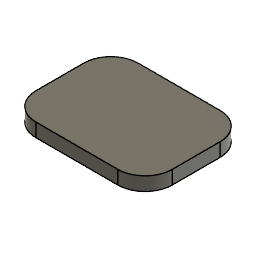
21_DAY- 3D Printable Mold (Autodesk Fusion 360 design; units mm, degrees)
part number: 2026-01-03-10-31-50-314
part number: 2026-01-03-10-33-35-516
part number: 2026-01-03-12-50-06-829
Autodesk Fusion 360 part; units mm, degrees
sketch "Sketch1" plane through (0, 0, 0) normal (0, 1, 0) x (1, 0, 0) in component "Key Chain"
  line L0 (0, 0) -> (50, 0)
  line L1 (50, 0) -> (50, 35)
  line L2 (50, 35) -> (0, 35)
  line L3 (0, 35) -> (0, 0)
  dimension "d1" = 50
  dimension "d2" = 35
  constraint horizontal L0
  constraint vertical L1
  constraint horizontal L2
  constraint vertical L3
  constraint coincident L0.start L3.end
  measures "d1" distance of L0.start L0.end
  measures "d2" distance of L0.start L2.end
extrude "Extrude1" add sketch "Sketch1" along normal blind 3 makes body 1 in component "Key Chain"
fillet "Fillet1" radius 7 4 edges at (0, 1.5, 0) (0, 1.5, -35) (50, 1.5, 0) (50, 1.5, -35) on bodies 1 in component "Key Chain"
sketch "Sketch2" plane through (0, 3, 0) normal (0, 1, 0) x (-1, 0, 0) in component "Key Chain"
  arc A0 (-50, -28) -> (-43, -35) centre (-43, -28) ccw
  line L0 (-43, -35) -> (-7, -35)
  arc A1 (-7, -35) -> (0, -28) centre (-7, -28) ccw
  line L1 (0, -28) -> (0, -7)
  arc A2 (0, -7) -> (-7, 0) centre (-7, -7) ccw
  line L2 (-7, 0) -> (-43, 0)
  arc A3 (-43, 0) -> (-50, -7) centre (-43, -7) ccw
  line L3 (-50, -7) -> (-50, -28)
  line L4 (-50, -17.5) -> (-45, -17.5) construction
  dimension "d7" = 5
  constraint midpoint L3 L4.start
  constraint perpendicular L3 L4
  measures "d7" distance of L4.start L4.end
hole "Hole1" at (45, 3, -17.5) direction (0, -1, 0) diameter 5 end up to surface (3 mm away) bodies 1 in component "Key Chain"
sketch "Sketch3" plane through (0, 3, 0) normal (0, 1, 0) x (-1, 0, 0) in component "Key Chain"
  circle A0 centre (-45, -17.5) radius 2.5
  arc A1 (-50, -28) -> (-43, -35) centre (-43, -28) ccw
  line L0 (-43, -35) -> (-7, -35)
  arc A2 (-7, -35) -> (0, -28) centre (-7, -28) ccw
  line L1 (0, -28) -> (0, -7)
  arc A3 (0, -7) -> (-7, 0) centre (-7, -7) ccw
  line L2 (-7, 0) -> (-43, 0)
  arc A4 (-43, 0) -> (-50, -7) centre (-43, -7) ccw
  line L3 (-50, -7) -> (-50, -28)
  line L4 (-3.7756, -4.293) -> (-42.3384, -4.293) construction
  line L5 (-42.3384, -4.293) -> (-42.3384, -31.526) construction
  line L6 (-42.3384, -31.526) -> (-3.7756, -31.526) construction
  line L7 (-3.7756, -31.526) -> (-3.7756, -4.293) construction
  dimension "d10" = 7
  text T0 "PIYUSH" font "Arial" height 7 bold align left middle in box 38.5628 x 27.233 at (-3.7756, -4.293) x (-1, 0) y (0, -1) spacing 1 kerned
extrude "Extrude2" add sketch "Sketch3" along normal blind 1 text T0 bodies 1 in component "Key Chain"
sketch "Sketch1 (2)" plane through (0, 3, 0) normal (0, 1, 0) x (-1, 0, 0) in component "One Part Mold"
  arc A0 (-50, -28) -> (-43, -35) centre (-43, -28) ccw
  line L0 (-43, -35) -> (-7, -35)
  arc A1 (-7, -35) -> (0, -28) centre (-7, -28) ccw
  line L1 (0, -28) -> (0, -7)
  arc A2 (0, -7) -> (-7, 0) centre (-7, -7) ccw
  line L2 (-7, 0) -> (-43, 0)
  arc A3 (-43, 0) -> (-50, -7) centre (-43, -7) ccw
  line L3 (-50, -7) -> (-50, -28)
  circle A4 centre (-45, -17.5) radius 2.5
  line L4 (-10.2551, -14.4095) -> (-10.2551, -21.4095)
  line L5 (-10.2551, -21.4095) -> (-11.6685, -21.4095)
  line L6 (-11.6685, -21.4095) -> (-11.6685, -14.4095)
  line L7 (-11.6685, -14.4095) -> (-10.2551, -14.4095)
  line L8 (-33.1269, -14.4095) -> (-33.1269, -21.4095)
  line L9 (-33.1269, -21.4095) -> (-34.5402, -21.4095)
  line L10 (-34.5402, -21.4095) -> (-34.5402, -18.6544)
  line L11 (-34.5402, -18.6544) -> (-37.3097, -18.6544)
  line L12 (-37.3097, -18.6544) -> (-37.3097, -21.4095)
  line L13 (-37.3097, -21.4095) -> (-38.723, -21.4095)
  line L14 (-38.723, -21.4095) -> (-38.723, -14.4095)
  line L15 (-38.723, -14.4095) -> (-37.3097, -14.4095)
  line L16 (-37.3097, -14.4095) -> (-37.3097, -17.4702)
  line L17 (-37.3097, -17.4702) -> (-34.5402, -17.4702)
  line L18 (-34.5402, -17.4702) -> (-34.5402, -14.4095)
  line L19 (-34.5402, -14.4095) -> (-33.1269, -14.4095)
  line L20 (-26.2415, -16.6871) -> (-27.6166, -16.8208)
  spline S0 degree 3 poles (-27.6166, -16.8208) (-27.6618, -16.6117) (-27.7446, -16.2287) (-28.0031, -15.9364) (-28.1204, -15.8038) knots 0 0 0 0 0.062919 0.115193 0.115193 0.115193 0.115193
  spline S1 degree 3 poles (-28.1204, -15.8038) (-28.2646, -15.7092) (-28.5745, -15.5059) (-28.946, -15.4884) (-29.1446, -15.4791) knots 0 0 0 0 0.050803 0.109205 0.109205 0.109205 0.109205
  spline S2 degree 3 poles (-29.1446, -15.4791) (-29.3497, -15.4847) (-29.7187, -15.4949) (-30.0337, -15.684) (-30.1736, -15.768) knots 0 0 0 0 0.060299 0.10848 0.10848 0.10848 0.10848
  spline S3 degree 3 poles (-30.1736, -15.768) (-30.2745, -15.8652) (-30.4678, -16.0515) (-30.503, -16.3168) (-30.5198, -16.4436) knots 0 0 0 0 0.040694 0.077943 0.077943 0.077943 0.077943
  spline S4 degree 3 poles (-30.5198, -16.4436) (-30.5143, -16.5225) (-30.5037, -16.6766) (-30.4166, -16.804) (-30.3741, -16.8662) knots 0 0 0 0 0.023266 0.045424 0.045424 0.045424 0.045424
  spline S5 degree 3 poles (-30.3741, -16.8662) (-30.31, -16.9245) (-30.1616, -17.0596) (-29.9728, -17.1296) (-29.8656, -17.1694) knots 0 0 0 0 0.025793 0.059689 0.059689 0.059689 0.059689
  spline S6 degree 3 poles (-29.8656, -17.1694) (-29.7302, -17.21) (-29.3558, -17.3223) (-28.9762, -17.4155) (-28.734, -17.475) knots 0 0 0 0 0.04242 0.117234 0.117234 0.117234 0.117234
  spline S7 degree 3 poles (-28.734, -17.475) (-28.4023, -17.5592) (-27.8316, -17.7042) (-27.3436, -18.0306) (-27.1391, -18.1673) knots 0 0 0 0 0.101661 0.174972 0.174972 0.174972 0.174972
  spline S8 degree 3 poles (-27.1391, -18.1673) (-26.9511, -18.3688) (-26.5795, -18.7671) (-26.5226, -19.3084) (-26.4945, -19.5759) knots 0 0 0 0 0.08029 0.15872 0.15872 0.15872 0.15872
  spline S9 degree 3 poles (-26.4945, -19.5759) (-26.5077, -19.7521) (-26.5342, -20.108) (-26.7093, -20.4191) (-26.7977, -20.5763) knots 0 0 0 0 0.0523 0.105673 0.105673 0.105673 0.105673
  spline S10 degree 3 poles (-26.7977, -20.5763) (-26.9126, -20.7233) (-27.1493, -21.0263) (-27.4941, -21.1973) (-27.6715, -21.2853) knots 0 0 0 0 0.055234 0.113816 0.113816 0.113816 0.113816
  spline S11 degree 3 poles (-27.6715, -21.2853) (-27.8796, -21.3563) (-28.3257, -21.5084) (-28.7974, -21.5217) (-29.0491, -21.5289) knots 0 0 0 0 0.065564 0.140598 0.140598 0.140598 0.140598
  spline S12 degree 3 poles (-29.0491, -21.5289) (-29.4455, -21.5172) (-30.1604, -21.4961) (-30.7641, -21.1191) (-31.0331, -20.9511) knots 0 0 0 0 0.116393 0.209938 0.209938 0.209938 0.209938
  spline S13 degree 3 poles (-31.0331, -20.9511) (-31.2288, -20.7385) (-31.6307, -20.302) (-31.6981, -19.7116) (-31.7326, -19.4088) knots 0 0 0 0 0.084432 0.173306 0.173306 0.173306 0.173306
  line L21 (-31.7326, -19.4088) -> (-30.3192, -19.3467)
  spline S14 degree 3 poles (-30.3192, -19.3467) (-30.2862, -19.5089) (-30.226, -19.8041) (-30.022, -20.0237) (-29.9301, -20.1227) knots 0 0 0 0 0.04852 0.088296 0.088296 0.088296 0.088296
  spline S15 degree 3 poles (-29.9301, -20.1227) (-29.8085, -20.1913) (-29.5321, -20.3474) (-29.2133, -20.3549) (-29.0348, -20.359) knots 0 0 0 0 0.041302 0.09386 0.09386 0.09386 0.09386
  spline S16 degree 3 poles (-29.0348, -20.359) (-28.8475, -20.3531) (-28.5055, -20.3423) (-28.2058, -20.1796) (-28.0703, -20.1059) knots 0 0 0 0 0.055275 0.100947 0.100947 0.100947 0.100947
  spline S17 degree 3 poles (-28.0703, -20.1059) (-28.0048, -20.0475) (-27.8746, -19.9312) (-27.8554, -19.7577) (-27.8458, -19.6714) knots 0 0 0 0 0.025368 0.050475 0.050475 0.050475 0.050475
  spline S18 degree 3 poles (-27.8458, -19.6714) (-27.8556, -19.5909) (-27.8756, -19.4249) (-27.9947, -19.3071) (-28.0559, -19.2465) knots 0 0 0 0 0.02363 0.048668 0.048668 0.048668 0.048668
  spline S19 degree 3 poles (-28.0559, -19.2465) (-28.2066, -19.1646) (-28.6141, -18.9431) (-29.0684, -18.8421) (-29.3547, -18.7785) knots 0 0 0 0 0.05125 0.138613 0.138613 0.138613 0.138613
  spline S20 degree 3 poles (-29.3547, -18.7785) (-29.6571, -18.7059) (-30.1801, -18.5804) (-30.6726, -18.3654) (-30.8803, -18.2748) knots 0 0 0 0 0.093065 0.16093 0.16093 0.16093 0.16093
  spline S21 degree 3 poles (-30.8803, -18.2748) (-31.0354, -18.1811) (-31.3416, -17.9963) (-31.5507, -17.7063) (-31.6538, -17.5633) knots 0 0 0 0 0.053748 0.106066 0.106066 0.106066 0.106066
  spline S22 degree 3 poles (-31.6538, -17.5633) (-31.7352, -17.3982) (-31.9082, -17.0473) (-31.9245, -16.6557) (-31.9331, -16.4484) knots 0 0 0 0 0.054613 0.11607 0.11607 0.11607 0.11607
  spline S23 degree 3 poles (-31.9331, -16.4484) (-31.9187, -16.2502) (-31.8896, -15.8503) (-31.6964, -15.4988) (-31.5989, -15.3215) knots 0 0 0 0 0.05885 0.118779 0.118779 0.118779 0.118779
  spline S24 degree 3 poles (-31.5989, -15.3215) (-31.4743, -15.157) (-31.2209, -14.8224) (-30.8447, -14.6357) (-30.6535, -14.5408) knots 0 0 0 0 0.061022 0.124107 0.124107 0.124107 0.124107
  spline S25 degree 3 poles (-30.6535, -14.5408) (-30.4265, -14.4664) (-29.9323, -14.3045) (-29.4118, -14.2921) (-29.1303, -14.2853) knots 0 0 0 0 0.071263 0.155186 0.155186 0.155186 0.155186
  spline S26 degree 3 poles (-29.1303, -14.2853) (-28.7274, -14.2998) (-27.9909, -14.3263) (-27.3718, -14.7204) (-27.0914, -14.8989) knots 0 0 0 0 0.118342 0.21636 0.21636 0.21636 0.21636
  spline S27 degree 3 poles (-27.0914, -14.8989) (-26.877, -15.1379) (-26.4192, -15.6484) (-26.3032, -16.3265) (-26.2415, -16.6871) knots 0 0 0 0 0.0944 0.201604 0.201604 0.201604 0.201604
  line L22 (-19.528, -21.4095) -> (-20.9413, -21.4095)
  line L23 (-20.9413, -21.4095) -> (-20.9413, -17.6182)
  spline S28 degree 3 poles (-20.9413, -17.6182) (-20.9399, -17.37) (-20.9375, -16.979) (-20.9788, -16.5903) (-20.9939, -16.4484) knots 0 0 0 0 0.074381 0.117178 0.117178 0.117178 0.117178
  spline S29 degree 3 poles (-20.9939, -16.4484) (-21.0342, -16.3125) (-21.1143, -16.0424) (-21.3225, -15.8527) (-21.426, -15.7584) knots 0 0 0 0 0.041663 0.082805 0.082805 0.082805 0.082805
  spline S30 degree 3 poles (-21.426, -15.7584) (-21.5575, -15.6827) (-21.8454, -15.5169) (-22.1786, -15.5047) (-22.3595, -15.4982) knots 0 0 0 0 0.044874 0.098214 0.098214 0.098214 0.098214
  spline S31 degree 3 poles (-22.3595, -15.4982) (-22.54, -15.5028) (-22.8639, -15.5111) (-23.1431, -15.6726) (-23.2667, -15.7441) knots 0 0 0 0 0.053119 0.095323 0.095323 0.095323 0.095323
  spline S32 degree 3 poles (-23.2667, -15.7441) (-23.3582, -15.8294) (-23.5374, -15.9966) (-23.6025, -16.2326) (-23.6344, -16.3481) knots 0 0 0 0 0.036734 0.071956 0.071956 0.071956 0.071956
  spline S33 degree 3 poles (-23.6344, -16.3481) (-23.6523, -16.5067) (-23.697, -16.9016) (-23.6966, -17.2992) (-23.6964, -17.5371) knots 0 0 0 0 0.047856 0.119139 0.119139 0.119139 0.119139
  line L24 (-23.6964, -17.5371) -> (-23.6964, -21.4095)
  line L25 (-23.6964, -21.4095) -> (-25.1098, -21.4095)
  line L26 (-25.1098, -21.4095) -> (-25.1098, -17.7328)
  spline S34 degree 3 poles (-25.1098, -17.7328) (-25.1104, -17.3736) (-25.1115, -16.777) (-25.0283, -16.1866) (-24.9952, -15.9518) knots 0 0 0 0 0.107593 0.178663 0.178663 0.178663 0.178663
  spline S35 degree 3 poles (-24.9952, -15.9518) (-24.9507, -15.7871) (-24.8643, -15.4677) (-24.6678, -15.2019) (-24.5726, -15.0732) knots 0 0 0 0 0.050679 0.098257 0.098257 0.098257 0.098257
  spline S36 degree 3 poles (-24.5726, -15.0732) (-24.4579, -14.9585) (-24.218, -14.7188) (-23.9098, -14.5767) (-23.749, -14.5026) knots 0 0 0 0 0.048273 0.100906 0.100906 0.100906 0.100906
  spline S37 degree 3 poles (-23.749, -14.5026) (-23.5523, -14.4408) (-23.1146, -14.3033) (-22.6553, -14.2948) (-22.4024, -14.2901) knots 0 0 0 0 0.061547 0.136938 0.136938 0.136938 0.136938
  spline S38 degree 3 poles (-22.4024, -14.2901) (-22.1058, -14.2929) (-21.5868, -14.2977) (-21.0932, -14.4545) (-20.8816, -14.5217) knots 0 0 0 0 0.088346 0.154588 0.154588 0.154588 0.154588
  spline S39 degree 3 poles (-20.8816, -14.5217) (-20.7205, -14.6016) (-20.4122, -14.7546) (-20.1757, -15.0042) (-20.0627, -15.1233) knots 0 0 0 0 0.053473 0.102324 0.102324 0.102324 0.102324
  spline S40 degree 3 poles (-20.0627, -15.1233) (-19.9716, -15.2457) (-19.7956, -15.4821) (-19.7085, -15.7635) (-19.6664, -15.8993) knots 0 0 0 0 0.045375 0.087695 0.087695 0.087695 0.087695
  spline S41 degree 3 poles (-19.6664, -15.8993) (-19.6263, -16.1471) (-19.5311, -16.7349) (-19.5291, -17.3308) (-19.528, -17.6755) knots 0 0 0 0 0.075209 0.178405 0.178405 0.178405 0.178405
  line L27 (-19.528, -17.6755) -> (-19.528, -21.4095)
  line L28 (-14.8533, -14.4095) -> (-14.8533, -17.3556)
  line L29 (-14.8533, -17.3556) -> (-12.2892, -21.4095)
  line L30 (-12.2892, -21.4095) -> (-13.9461, -21.4095)
  line L31 (-13.9461, -21.4095) -> (-15.5934, -18.6401)
  line L32 (-15.5934, -18.6401) -> (-17.2074, -21.4095)
  line L33 (-17.2074, -21.4095) -> (-18.8356, -21.4095)
  line L34 (-18.8356, -21.4095) -> (-16.2619, -17.3461)
  line L35 (-16.2619, -17.3461) -> (-16.2619, -14.4095)
  line L36 (-16.2619, -14.4095) -> (-14.8533, -14.4095)
  line L37 (-3.7756, -14.4095) -> (-3.7756, -21.4095)
  line L38 (-3.7756, -21.4095) -> (-6.0436, -21.4095)
  spline S42 degree 3 poles (-6.0436, -21.4095) (-6.3995, -21.4122) (-6.9627, -21.4165) (-7.5194, -21.3346) (-7.7244, -21.3044) knots 0 0 0 0 0.106513 0.168611 0.168611 0.168611 0.168611
  spline S43 degree 3 poles (-7.7244, -21.3044) (-7.918, -21.2349) (-8.3124, -21.0933) (-8.5904, -20.7792) (-8.7319, -20.6192) knots 0 0 0 0 0.060664 0.123606 0.123606 0.123606 0.123606
  spline S44 degree 3 poles (-8.7319, -20.6192) (-8.8502, -20.4229) (-9.1021, -20.0045) (-9.1254, -19.5155) (-9.1378, -19.256) knots 0 0 0 0 0.067692 0.144229 0.144229 0.144229 0.144229
  spline S45 degree 3 poles (-9.1378, -19.256) (-9.1309, -19.0554) (-9.1181, -18.6795) (-8.972, -18.3335) (-8.9038, -18.1721) knots 0 0 0 0 0.059616 0.111721 0.111721 0.111721 0.111721
  spline S46 degree 3 poles (-8.9038, -18.1721) (-8.8226, -18.035) (-8.6654, -17.7695) (-8.4254, -17.5758) (-8.3093, -17.4821) knots 0 0 0 0 0.047362 0.091731 0.091731 0.091731 0.091731
  spline S47 degree 3 poles (-8.3093, -17.4821) (-8.1911, -17.4062) (-7.9629, -17.2596) (-7.7021, -17.1858) (-7.5764, -17.1503) knots 0 0 0 0 0.041895 0.080851 0.080851 0.080851 0.080851
  spline S48 degree 3 poles (-7.5764, -17.1503) (-7.3702, -17.1212) (-6.8842, -17.0527) (-6.3932, -17.051) (-6.1105, -17.05) knots 0 0 0 0 0.062409 0.147081 0.147081 0.147081 0.147081
  line L39 (-6.1105, -17.05) -> (-5.1889, -17.05)
  line L40 (-5.1889, -17.05) -> (-5.1889, -14.4095)
  line L41 (-5.1889, -14.4095) -> (-3.7756, -14.4095)
  line L42 (5, -28) -> (5, -7)
  arc A5 (5, -7) -> (-7, 5) centre (-7, -7) ccw
  line L43 (-7, 5) -> (-43, 5)
  arc A6 (-43, 5) -> (-55, -7) centre (-43, -7) ccw
  line L44 (-55, -7) -> (-55, -28)
  arc A7 (-55, -28) -> (-43, -40) centre (-43, -28) ccw
  line L45 (-43, -40) -> (-7, -40)
  arc A8 (-7, -40) -> (5, -28) centre (-7, -28) ccw
  dimension "d14" = 5
extrude "Extrude1'" add sketch "Sketch1 (2)" along normal blind 6 separate body contours A0 L0 A1 L1 A2 L2 A3 L3 | A4 | L4 L5 L6 L7 | L8 L9 L10 L11 L12 L13 L14 L15 L16 L17 L18 L19 | L20 S0 S1 S2 S3 S4 S5 S6 S7 S8 S9 S10 S11 S12 S13 L21 S14 S15 S16 S17 S18 S19 S20 S21 S22 S23 S24 S25 S26 S27 | L22 L23 S28 S29 S30 S31 S32 S33 L24 L25 L26 S34 S35 S36 S37 S38 S39 S40 S41 L27 | L28 L29 L30 L31 L32 L33 L34 L35 L36 | L37 L38 S42 S43 S44 S45 S46 S47 S48 L39 L40 L41 | L42 A5 L43 A6 L44 A7 L45 A8 makes body 2 in component "One Part Mold"
combine "Combine1" operation cut target body 2 tool bodies 1 keep tools in component "One Part Mold"
draft "Draft1" angle 5 neutral plane through (0, 3, 0) pull (0, -1, 0) 8 faces at (31, 1, -35) (49.9921, 1, -28.3331) (50, 1, -14) (43.3331, 1, -0.0079) (19, 2, 0) (6.6669, 1, -0.0079) (0, 1, -21) (6.6669, 1, -34.9921) on bodies 1 in component "Key Chain"
draft "Draft2" angle -5 neutral plane through (0, 0, 0) pull (0, -1, 0) 1 faces at (45.1246, 2, -15.0031) on bodies 1 in component "Key Chain"
component "Key Chain" placed x (1, 0, 0) y (0, 1, 0) z (0, 0, 1) at (0, 0, 0)
component "One Part Mold" placed x (1, 0, 0) y (0, 1, 0) z (0, 0, 1) at (0, 0, 0) in component "Key Chain"
equation "d11 = 'PIYUSH'"
